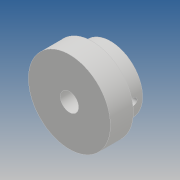
# Autodesk Inventor part: poleaT5
Saved by Autodesk Inventor 2017 (Build 210142000, 142)
## iProperties
Part Number: poleaT5
Material: Genérico
Document SubType Name: Modeling
Designer: Leo
Density: 1 g/cm^3
Appearance: Valor por defecto
Author: Leo
Autodesk Inventor part; units mm, degrees
ref_plane "YZ Plane" through (0, 0, 0) normal (1, 0, 0) x (0, 1, 0)
ref_plane "XZ Plane" through (0, 0, 0) normal (0, 1, 0) x (-1, 0, 0)
ref_plane "XY Plane" through (0, 0, 0) normal (0, 0, 1) x (1, 0, 0)
sketch "Boceto1" plane through (0, 0, 0) normal (0, 1, 0) x (-1, 0, 0)
  circle A0 centre (0, 0) radius 4
  circle A1 centre (0, 0) radius 14
  line L0 (-7.0696, 2.75) -> (-10.0696, 2.75)
  line L1 (-10.0696, 2.75) -> (-10.0696, -2.75)
  line L2 (-10.0696, -2.75) -> (-7.0696, -2.75)
  line L3 (-7.0696, -2.75) -> (-7.0696, 2.75)
  circle A2 centre (0, 0) radius 9 construction
  point P0 (-7.0696, 0)
  point P1 (-8.5696, 2.75)
  dimension "d0" = 8
  dimension "tuerca" = 5.5
  dimension "d2" = 10
  dimension "d3" = 5
  dimension "d4" = 3
  constraints: 8 end point, 2 centre point, 2 coincident, 2 midpoint, 2 parallel, 1 horizontal, 1 horizontal alignment, 1 perpendicular, 3 other
  measures "d0" diameter of A0
  measures "tuerca" distance of L0.end L1.end
  measures "d2" radial gap between concentric circles of A1 A0
  measures "d4" distance of L0.start L0.end
extrude "Extrusión1" add sketch "Boceto1" along normal blind 8
sketch "Boceto2" plane through (7.0696, 0, -2.75) normal (1, 0, 0) x (0, 0, -1)
  line L0 (0, 0) -> (-5.5, 0) projected
  line L1 (0, 0) -> (0, 8) construction
  line L2 (-5.5, 8) -> (0, 8) construction
  line L3 (-5.5, 0) -> (-5.5, 8) construction
  line L4 (-5.5, 0) -> (0, 8) construction
  circle A0 centre (-2.75, 4) radius 1.6
  line L5 (0, 2.1813) -> (-2.75, 0.5936)
  line L6 (-2.75, 0.5936) -> (-5.5, 2.1813)
  line L7 (-5.5, 2.1813) -> (-5.5, 0)
  line L8 (0, 2.1813) -> (0, 0)
  point P0 (-2.75, 0)
  dimension "d7" = 3.2
  dimension "d8" = 120
  dimension "d9" = 2.95
  constraints: 10 end point, 2 point on line, 1 centre point, 1 collinear, 1 equal length, 1 horizontal alignment, 1 midpoint
  measures "d7" diameter of A0
  measures "d8" angle of L5 L6
  measures "d9" distance from line of A0.centre L5
extrude "Extrusión2" cut sketch "Boceto2" along normal mid plane 15 contours A0
extrude "Extrusión3" add sketch "Boceto2" along normal up to next contours L0 L7 L6 L5 L8
sketch "Boceto3" plane through (0, 0, 0) normal (0, -1, 0) x (1, 0, 0)
  circle A0 centre (0, 0) radius 4 projected
  circle A1 centre (0, 0) radius 17.939
  constraints: 1 centre point
extrude "Extrusión4" add sketch "Boceto3" along normal blind 10
equation "\"d3\" = 0.5 * d2"
